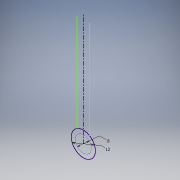
# Autodesk Inventor part: Arm1
Saved by Autodesk Inventor 2019 (Build 230136000, 136)
## iProperties
Created: 2021-01-08
Part Number: Arm1
Material: Generic
Document SubType Name: Modeling
Designer: Sam
Density: 1 g/cm^3
Appearance: Default
Author: Sam
Autodesk Inventor part; units mm, degrees
ref_plane "YZ Plane" through (0, 0, 0) normal (1, 0, 0) x (0, 1, 0)
ref_plane "XZ Plane" through (0, 0, 0) normal (0, 1, 0) x (-1, 0, 0)
ref_plane "XY Plane" through (0, 0, 0) normal (0, 0, 1) x (1, 0, 0)
sketch "Sketch1" plane through (0, 0, 0) normal (0, 0, 1) x (1, 0, 0)
  circle A0 centre (0, 0) radius 4 construction
  arc A1 (-4, 5.7446) -> (4, 5.7446) centre (0, 0) ccw
  line L0 (0, 0) -> (0, 55.7184)
  line L1 (4, 5.7446) -> (4, 73)
  line L2 (-4, 5.7446) -> (-4, 73)
  line L3 (-6, 87) -> (6, 87)
  line L4 (6, 87) -> (6, 73)
  line L5 (-6, 73) -> (-6, 87)
  line L6 (11.9426, 80) -> (-16.3148, 80) construction
  line L7 (6, 73) -> (4, 73)
  line L8 (-4, 73) -> (-6, 73)
  arc A2 (1.118, -1) -> (-1.118, -1) centre (0, 0) ccw
  line L9 (1.118, -1) -> (-1.118, -1)
  circle A3 centre (0, 80) radius 2.05
  dimension "d0" = 8
  dimension "d1" = 14
  dimension "d2" = 8
  dimension "d3" = 12
  dimension "d4" = 14
  dimension "d6" = 80
  dimension "d7" = 3
  dimension "d8" = 1
  dimension "d9" = 4.1
  constraints: 20 end point, 4 centre point, 4 point on circle, 3 horizontal, 3 parallel, 3 vertical, 2 coincident, 1 collinear, 1 perpendicular, 1 point on line, 1 vertical alignment, 3 other
  measures "d0" diameter of A0
  measures "d1" diameter of A1
  measures "d2" distance between parallel lines of L2 L1
  measures "d3" distance of L3.start L3.end
  measures "d4" distance of L5.start L3.start
  measures "d6" distance from line of point (0, 0) L6
  measures "d7" diameter of A2
  measures "d8" distance from line of L9 point (0, 0)
  measures "d9" diameter of A3
extrude "Extrusion1" add sketch "Sketch1" along normal blind 8
sketch "Sketch2" plane through (0, 0, 0) normal (0, 0, -1) x (-1, 0, 0)
  circle A0 centre (0, 0) radius 4.05
  dimension "d12" = 8.1
  constraints: 1 centre point, 1 coincident
  measures "d12" diameter of A0
extrude "Extrusion2" cut sketch "Sketch2" against normal blind 1.5
sketch "Sketch3" plane through (0, 0, 0) normal (0, 0, -1) x (-1, 0, 0)
  line L0 (-4, 73) -> (-4, 5.7446) projected
  line L1 (4, 5.7446) -> (4, 73) projected
  arc A0 (4, 5.7446) -> (-4, 5.7446) centre (0, 0) ccw
  line L2 (4, 73) -> (6, 73) projected
  line L3 (-4, 73) -> (4, 73)
  constraints: 4 end point, 2 point on circle, 1 centre point, 1 coincident, 1 horizontal
extrude "Extrusion3" cut sketch "Sketch3" against normal blind 3
sketch "Sketch4" plane through (0, 0, 0) normal (0, 0, -1) x (-1, 0, 0)
  line L0 (-6, 73) -> (-6, 87) projected
  line L1 (6, 87) -> (6, 73) projected
  line L2 (-6, 75) -> (6, 75)
  line L3 (6, 75) -> (6, 85)
  line L4 (6, 85) -> (-6, 85)
  line L5 (-6, 85) -> (-6, 75)
  line L6 (-6, 73) -> (6, 73) projected
  line L7 (6, 87) -> (-6, 87) projected
  point P0 (0, 0)
  dimension "d17" = 2
  dimension "d18" = 2
  constraints: 8 end point, 2 parallel, 2 point on line, 1 horizontal, 1 perpendicular
  measures "d17" distance between parallel lines of L6 L2
  measures "d18" distance between parallel lines of L7 L4
extrude "Extrusion4" cut sketch "Sketch4" against normal blind 6 contours L0 L4 L1 L2
fillet "Fillet1" radius 1 6 edges at (4, 73, 5.5) (0, 73, 3) (-4, 73, 5.5) (0, 7, 3) (4, 5.7446, 5.5) (-4, 5.7446, 5.5)
sketch "Sketch5" plane through (0, 0, 6) normal (0, 0, -1) x (-1, 0, 0)
  circle A0 centre (-4.5, 80) radius 0.6105 projected
  circle A1 centre (4.5, 80) radius 0.6105 projected
  circle A2 centre (-4.5, 80) radius 0.5
  circle A3 centre (4.5, 80) radius 0.5
  point P0 (0, 0)
  dimension "d22" = 1
  constraints: 2 centre point, 2 coincident, 1 equal radius
  measures "d22" diameter of A2
extrude "Extrusion5" add sketch "Sketch5" along normal blind 2 contours A2 | A3
fillet "Fillet2" radius 0.1 2 edges at (5, 80, 6) (-4, 80, 6)
fillet "Fillet3" radius 0.4 2 edges at (5, 80, 4) (-4, 80, 4)
body "Solid1"
